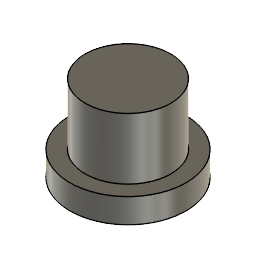
Button_Stub (Autodesk Fusion 360 design; units mm, degrees)
Autodesk Fusion 360 part; units mm, degrees
sketch "Sketch1" plane through (0, 0, 0) normal (0, 0, 1) x (1, 0, 0)
  circle A0 centre (0, 0) radius 1.9
  dimension "d1" = 3.8
  constraint coincident A0.centre origin
  measures "d1" diameter of A0
extrude "Extrude1" add sketch "Sketch1" along normal blind 0.8
sketch "Sketch2" plane through (0, 0, 0.8) normal (0, 0, 1) x (-1, 0, 0)
  circle A0 centre (0, 0) radius 1.9
  circle A1 centre (0, 0) radius 1.4
  dimension "d4" = 2.8
  constraint coincident A0.centre A1.centre
  measures "d4" diameter of A1
extrude "Extrude2" add sketch "Sketch2" along normal blind 1 contours A1
extrude "Extrude3" add 1 faces at (-0.5498, 0.3174, 1.8) along direction (0, 0, 1) blind 1
